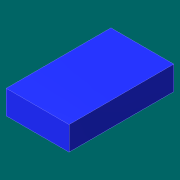
# Autodesk Inventor part: mppcMountClamp
Saved by Autodesk Inventor 2016 (Build 200138000, 138)
## iProperties
Created: 2016-02-18
Part Number: mppcMountClamp
Material: ABS Plastic
Document SubType Name: Modeling
Designer: Sawaiz
Density: 1.06 g/cm^3
Appearance: Blue - Wall Paint - Glossy
Author: Sawaiz
Autodesk Inventor part; units mm, degrees
ref_plane "YZ Plane" through (0, 0, 0) normal (1, 0, 0) x (0, 1, 0)
ref_plane "XZ Plane" through (0, 0, 0) normal (0, 1, 0) x (-1, 0, 0)
ref_plane "XY Plane" through (0, 0, 0) normal (0, 0, 1) x (1, 0, 0)
sketch "Sketch1" plane through (0, 0, 0) normal (0, 0, 1) x (1, 0, 0)
  line L0 (12.5, 7.5) -> (-12.5, 7.5)
  line L1 (-12.5, 7.5) -> (-12.5, -7.5)
  line L2 (-12.5, -7.5) -> (12.5, -7.5)
  line L3 (12.5, -7.5) -> (12.5, 7.5)
  line L4 (12.5, 7.5) -> (-12.5, -7.5) construction
  line L5 (-12.5, 7.5) -> (12.5, -7.5) construction
  point P0 (0, 0)
  dimension "d0" = 25
  dimension "d1" = 15
  constraints: 12 end point, 2 midpoint, 2 parallel, 1 horizontal, 1 perpendicular
  measures "d0" distance of L1.end L2.end
  measures "d1" distance between parallel lines of L0 L2
extrude "Extrusion1" add sketch "Sketch1" along normal blind 5.7
equation "\"d1\" = mppcMountDepth"
equation "\"d2\" = rubberizedCoating + 0.5 * ScintillatorWidth + silveringThickness"
equation "\"silveringThickness\" = 0.2"
equation "\"rubberizedCoating\" = 0.5"
equation "\"OpticalFiberClearence\" = 0.1"
equation "\"ScintillatorEdgeClearence\" = 3"
equation "\"ShallowTrackDepth\" = 1.2"
equation "\"DeepTrackDepth\" = 5.6"
equation "\"FiberEdgeOffsett\" = 5"
equation "\"LoopLargeTrackRatio\" = 1.1"
equation "\"FiberSensorClerence\" = 0.5"
equation "\"MountingScrewOffsett\" = 9"
equation "\"mppcMountDepth\" = 15"
equation "\"ScintillatorWidth\" = 10"
body "Solid1"
